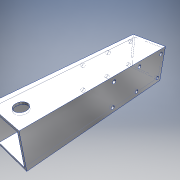
# Autodesk Inventor part: Arm 18 inch
Saved by Autodesk Inventor 2019 (Build 230136000, 136)
## iProperties
Created: 2018-09-22
Part Number: Arm 18 inch
Material: Aluminum 6061
Document SubType Name: Modeling
Designer: Adhik
Density: 2.7 g/cm^3
Appearance: Aluminum - Flat
Mass: 369.322 g
Surface Area: 881.709 cm^2
Volume: 136.786 cm^3
Author: Adhik
Autodesk Inventor part; units mm, degrees
ref_plane "YZ Plane" through (0, 0, 0) normal (1, 0, 0) x (0, 1, 0)
ref_plane "XZ Plane" through (0, 0, 0) normal (0, 1, 0) x (-1, 0, 0)
ref_plane "XY Plane" through (0, 0, 0) normal (0, 0, 1) x (1, 0, 0)
sketch "Sketch1" plane through (0, 0, 0) normal (0, 0, 1) x (1, 0, 0)
  line L0 (-35.56, 0) -> (35.56, 0) construction
  line L1 (0, -35.56) -> (0, 35.56) construction
  line L2 (-25.4, 25.4) -> (25.4, 25.4)
  line L3 (25.4, 25.4) -> (25.4, -25.4)
  line L4 (25.4, -25.4) -> (-25.4, -25.4)
  line L5 (-25.4, -25.4) -> (-25.4, 25.4)
  line L6 (-22.225, 22.225) -> (22.225, 22.225)
  line L7 (22.225, 22.225) -> (22.225, -22.225)
  line L8 (22.225, -22.225) -> (-22.225, -22.225)
  line L9 (-22.225, -22.225) -> (-22.225, 22.225)
  point P0 (0, 0)
  point P1 (-25.4, 0)
  point P2 (0, 25.4)
  point P3 (-22.225, 0)
  point P4 (0, 22.225)
  dimension "d0" = 50.8
  dimension "d1" = 3.175
  constraints: 16 end point, 4 midpoint, 4 parallel, 4 perpendicular, 4 point on line, 2 horizontal
  measures "d0" distance of L4.end L2.start
  measures "d1" distance between parallel lines of L2 L6
extrude "Extrusion1" add sketch "Sketch1" along normal mid plane 215.9
sketch "Sketch2" plane through (25.4, -25.4, 107.95) normal (1, 0, 0) x (0, 0, -1)
  line L0 (268.3764, 25.4) -> (-44.7294, 25.4) construction
  line L1 (107.95, -10.16) -> (107.95, 60.96) construction
  line L2 (119.38, 7.62) -> (208.28, 7.62) construction
  line L3 (208.28, 7.62) -> (208.28, 43.18) construction
  line L4 (208.28, 43.18) -> (119.38, 43.18) construction
  line L5 (119.38, 43.18) -> (119.38, 7.62) construction
  circle A0 centre (119.38, 43.18) radius 2.667
  circle A1 centre (119.38, 7.62) radius 2.667
  circle A2 centre (163.83, 7.62) radius 2.667
  circle A3 centre (208.28, 7.62) radius 2.667
  circle A4 centre (208.28, 43.18) radius 2.667
  circle A5 centre (163.83, 43.18) radius 2.667
  line L6 (215.9, 50.8) -> (215.9, 0) construction
  point P0 (107.95, 25.4)
  point P1 (208.28, 25.4)
  dimension "d4" = 5.334
  dimension "d5" = 7.62
  dimension "d6" = 88.9
  dimension "d7" = 17.78
  constraints: 8 end point, 6 centre point, 5 equal radius, 4 coincident, 3 midpoint, 2 parallel, 1 horizontal, 1 perpendicular, 1 point on line
  measures "d4" diameter of A1
  measures "d5" distance between parallel lines of L6 L3
  measures "d6" distance of L3.end L4.end
  measures "d7" distance between parallel lines of L0 L4
extrude "Extrusion2" cut sketch "Sketch2" against normal through all
sketch "Sketch4" plane through (-25.4, 25.4, 107.95) normal (0, 1, 0) x (1, 0, 0)
  line L0 (25.4, 259.08) -> (25.4, -43.18) construction
  line L1 (-10.16, 107.95) -> (60.96, 107.95) construction
  circle A0 centre (25.4, 19.05) radius 7.9375
  line L2 (50.8, 0) -> (0, 0) construction
  line L3 (38.1, 6.35) -> (12.7, 6.35) construction
  line L4 (12.7, 6.35) -> (12.7, 31.75) construction
  line L5 (12.7, 31.75) -> (38.1, 31.75) construction
  line L6 (38.1, 31.75) -> (38.1, 6.35) construction
  line L7 (38.1, 19.05) -> (12.7, 19.05) construction
  circle A1 centre (38.1, 6.35) radius 2.413 construction
  circle A2 centre (12.7, 6.35) radius 2.413 construction
  circle A3 centre (12.7, 31.75) radius 2.413 construction
  circle A4 centre (38.1, 31.75) radius 2.413 construction
  point P0 (25.4, 107.95)
  point P1 (25.4, 6.35)
  dimension "d13" = 15.875
  dimension "d14" = 19.05
  dimension "d17" = 4.826
  dimension "d18" = 25.4
  constraints: 10 end point, 5 centre point, 4 coincident, 4 midpoint, 3 equal radius, 2 horizontal, 2 parallel, 2 perpendicular, 2 point on line
  measures "d13" diameter of A0
  measures "d14" distance from line of A0.centre L2
  measures "d17" diameter of A1
  measures "d18" distance of L5.end L3.start
extrude "Extrusion6" cut sketch "Sketch4" against normal up to next
body "Solid1"
